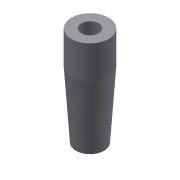
# Autodesk Inventor part: Vented_plug
Saved by Autodesk Inventor 2014 (Build 180170000, 170)
## iProperties
Created: 2016-08-28
Part Number: Vented_plug
Material: Generic
Document SubType Name: Modeling
Designer: Camilo
Density: 1 g/cm^3
Appearance: Default
Author: Camilo
Autodesk Inventor part; units mm, degrees
ref_plane "YZ Plane" through (0, 0, 0) normal (1, 0, 0) x (0, 1, 0)
ref_plane "XZ Plane" through (0, 0, 0) normal (0, 1, 0) x (-1, 0, 0)
ref_plane "XY Plane" through (0, 0, 0) normal (0, 0, 1) x (1, 0, 0)
sketch "Sketch1" plane through (0, 0, 0) normal (0, 0, 1) x (1, 0, 0)
  circle A0 centre (0, 0) radius 7.94 construction
  circle A1 centre (0, 0) radius 8.44
  point P0 (0, 0)
  dimension "d5" = 0.5
  constraints: 1 centre point, 1 coincident
  measures "d5" radial gap between concentric circles of A0 A1
extrude "Extrusion1" add sketch "Sketch1" along normal blind 10 and the other way blind 20
sketch "Sketch2" plane through (0, 0, 0) normal (1, 0, 0) x (0, 1, 0)
  line L0 (-8.44, -20) -> (8.44, -20) construction
  line L1 (8.44, 10) -> (-8.44, 10) construction
  line L2 (8.44, 10) -> (8.44, -20)
  line L3 (8.44, 10) -> (6.44, -20)
  line L4 (8.44, -20) -> (6.44, -20)
  line L5 (0, -26) -> (0, 16) projected
  point P0 (0, 0)
  dimension "d6" = 2
  constraints: 6 end point, 1 point on line
  measures "d6" distance of L0.end L3.end
revolve "Revolution1" cut sketch "Sketch2" angle 360 about axis through (0, 0, 10) along (0, 0, 1)
sketch "Sketch3" plane through (0, 0, -20) normal (0, 0, -1) x (-1, 0, 0)
  circle A0 centre (0, 0) radius 6.44 construction
  circle A1 centre (0, 0) radius 3.94
  dimension "d8" = 2.5
  constraints: 1 centre point, 1 coincident
  measures "d8" radial gap between concentric circles of A0 A1
extrude "Extrusion2" cut sketch "Sketch3" against normal through all
sketch "Sketch4" plane through (0, 0, 10) normal (0, 0, 1) x (1, 0, 0)
  circle A0 centre (0, 0) radius 3.94 projected
  circle A1 centre (0, 0) radius 8.44 projected
extrude "Extrusion3" add sketch "Sketch4" along normal blind 15
body "Solid1"
